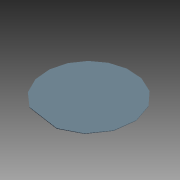
# Autodesk Inventor part: combdrive-test
Saved by Autodesk Inventor 2011 SP1 (Build 150282100, 282)
## iProperties
Created: 2011-03-23
Part Number: combdrive-test
Document SubType Name: Modeling
Designer: Andrew Zonenberg
Density: 2.329 g/cm^3
Material: Silicon
Mass: 9.53097 g
Surface Area: 157.543 cm^2
Volume: 4.0923 cm^3
Author: Andrew Zonenberg
Autodesk Inventor part; units mm, degrees
ref_plane "YZ Plane" through (0, 0, 0) normal (1, 0, 0) x (0, 1, 0)
ref_plane "XZ Plane" through (0, 0, 0) normal (0, 1, 0) x (-1, 0, 0)
ref_plane "XY Plane" through (0, 0, 0) normal (0, 0, 1) x (1, 0, 0)
sketch "Sketch1" plane through (0, 0, 0) normal (0, 0, 1) x (1, 0, 0)
  circle A0 centre (0, 0) radius 50
  line L0 (-16.25, -47.2857) -> (16.25, -47.2857)
  dimension "d1" = 32.5
  dimension "d2" = 100
  constraints: 2 end point, 2 point on circle, 1 centre point, 1 coincident, 1 horizontal
  measures "d1" distance of L0.end L0.start
  measures "d2" diameter of A0
extrude "Extrusion1" add sketch "Sketch1" along normal blind 0.525 contours A0 L0 picked at (-0.3738, -14.8613)
sketch "Sketch2" plane through (0, 0, 0.525) normal (0, 0, 1) x (1, 0, 0)
  arc A0 (16.25, -47.2857) -> (-16.25, -47.2857) centre (0, 0) ccw projected
  line L0 (-0.35, 0.35) -> (-0.3, 0.35)
  line L1 (-0.3, 0.35) -> (-0.3, 0.3)
  line L2 (-0.3, 0.3) -> (-0.25, 0.3)
  line L3 (-0.25, 0.3) -> (-0.25, 0.25)
  line L4 (-0.25, 0.25) -> (-0.3, 0.25)
  line L5 (-0.3, 0.25) -> (-0.3, 0.2)
  line L6 (-0.3, 0.2) -> (-0.35, 0.2)
  line L7 (-0.35, 0.2) -> (-0.35, 0.25)
  line L8 (-0.35, 0.25) -> (-0.4, 0.25)
  line L9 (-0.4, 0.25) -> (-0.4, 0.3)
  line L10 (-0.4, 0.3) -> (-0.35, 0.3)
  line L11 (-0.35, 0.3) -> (-0.35, 0.35)
  dimension "d5" = 0.05
  dimension "d6" = 0.25
  dimension "d7" = 0.25
  constraints: 24 end point, 11 equal length, 8 perpendicular, 1 vertical
  measures "d5" distance between parallel lines of L8 L10
  measures "d6" distance from line of L3 A0.centre
  measures "d7" distance from line of A0.centre L4
extrude "Extrusion2" cut sketch "Sketch2" against normal blind 0.025
chamfer "Chamfer2" distance 0.0249 angle 35.3 12 edges at (-0.325, 0.35, 0.5) (-0.35, 0.325, 0.5) (-0.375, 0.3, 0.5) (-0.4, 0.275, 0.5) (-0.375, 0.25, 0.5) (-0.35, 0.225, 0.5) (-0.325, 0.2, 0.5) (-0.3, 0.225, 0.5) (-0.275, 0.25, 0.5) (-0.25, 0.275, 0.5) (-0.275, 0.3, 0.5) (-0.3, 0.325, 0.5) measured on face at (-0.3833, 0.2833, 0.5)
body "Solid1"
